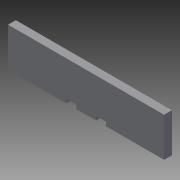
# Autodesk Inventor part: castlegen
Saved by Autodesk Inventor 2014 (Build 180170000, 170)
## iProperties
Created: 2014-07-15
Part Number: castlegen
Material: Generic
Document SubType Name: Modeling
Designer: cruiser
Density: 1 g/cm^3
Appearance: Default
Author: cruiser
Autodesk Inventor part; units mm, degrees
ref_plane "YZ Plane" through (0, 0, 0) normal (1, 0, 0) x (0, 1, 0)
ref_plane "XZ Plane" through (0, 0, 0) normal (0, 1, 0) x (-1, 0, 0)
ref_plane "XY Plane" through (0, 0, 0) normal (0, 0, 1) x (1, 0, 0)
sketch "Sketch1" plane through (0, 0, 0) normal (0, 1, 0) x (-1, 0, 0)
  line L0 (100, -25) -> (-100, -25)
  line L1 (-100, -25) -> (-100, 25)
  line L2 (-100, 25) -> (100, 25)
  line L3 (100, 25) -> (100, -25)
  line L4 (100, -25) -> (-100, 25) construction
  line L5 (-100, -25) -> (100, 25) construction
  point P0 (0, 0)
  dimension "d0" = 200
  dimension "d1" = 50
  constraints: 12 end point, 2 midpoint, 2 parallel, 1 horizontal, 1 perpendicular
  measures "d0" distance of L1.end L2.end
  measures "d1" distance of L0.end L1.end
extrude "Extrusion1" add sketch "Sketch1" along normal blind 10
sketch "Sketch2" plane through (0, 10, 0) normal (0, 1, 0) x (1, 0, 0)
  line L0 (100, 25) -> (-100, 25) projected
  line L1 (0, 0) -> (0, 25)
  line L2 (-12.7, 25) -> (-25.4, 25)
  line L3 (-25.4, 25) -> (-25.4, 19.92)
  line L4 (-25.4, 19.92) -> (-12.7, 19.92)
  line L5 (-12.7, 19.92) -> (-12.7, 25)
  line L6 (12.7, 25) -> (25.4, 25)
  line L7 (25.4, 25) -> (25.4, 19.92)
  line L8 (25.4, 19.92) -> (12.7, 19.92)
  line L9 (12.7, 19.92) -> (12.7, 25)
  dimension "d5" = 5.08
  dimension "d6" = 25.4
  dimension "d9" = 5.08
  dimension "d12" = 50.8
  constraints: 18 end point, 4 parallel, 2 horizontal, 2 perpendicular, 2 point on line, 1 coincident, 1 midpoint, 2 other
  measures "d5" distance between parallel lines of L8 L0
  measures "d6" distance between parallel lines of L5 L9
  measures "d9" distance of L2.end L3.end
  measures "d12" distance between parallel lines of L3 L7
extrude "Extrusion2" cut sketch "Sketch2" against normal up to next
equation "\"d5\" = m2_thickness"
equation "\"d6\" = castle_width"
equation "\"d9\" = m2_thickness"
equation "\"d12\" = castle_pitch"
equation "\"m2_thickness\" = 5.08"
equation "\"castle_width\" = 25.4"
equation "\"castle_pitch\" = 50.8"
body "Solid1"
